Autodesk Inventor part; units mm, degrees
(part 2 of 4)
  arc A608 (10.5835, 25.1123) -> (10.4066, 24.8539) centre (14.8434, 22.0065) ccw
  arc A609 (10.8252, 25.4234) -> (10.5835, 25.1123) centre (15.7615, 21.3378) ccw
  arc A610 (11.147, 25.7878) -> (10.8252, 25.4234) centre (16.6706, 20.5861) ccw
  arc A611 (9.9958, 26.1618) -> (9.6113, 26.2702) centre (4.2393, 6.4866) ccw
  arc A612 (10.0419, 25.6779) -> (9.9958, 26.1618) centre (2.4697, 25.2002) ccw
  arc A613 (10.0547, 25.2841) -> (10.0419, 25.6779) centre (3.647, 25.2741) ccw
  arc A614 (10.4066, 24.8539) -> (10.0459, 24.9711) centre (4.2393, 6.4866) ccw
  arc A615 (10.0459, 24.9711) -> (10.0547, 25.2841) centre (4.7827, 25.2754) ccw
  arc A616 (9.1026, 25.5526) -> (8.9465, 25.2811) centre (13.5931, 22.7906) ccw
  arc A617 (9.3192, 25.8817) -> (9.1026, 25.5526) centre (14.5608, 22.1961) ccw
  arc A618 (9.6113, 26.2702) -> (9.3192, 25.8817) centre (15.526, 21.5179) ccw
  arc A619 (8.4344, 26.5528) -> (8.0426, 26.6307) centre (4.2393, 6.4866) ccw
  arc A620 (8.5183, 26.074) -> (8.4344, 26.5528) centre (1.0069, 25.0037) ccw
  arc A621 (8.5619, 25.6824) -> (8.5183, 26.074) centre (2.1747, 25.1697) ccw
  arc A622 (8.9465, 25.2811) -> (8.5777, 25.3697) centre (4.2393, 6.4866) ccw
  arc A623 (8.5777, 25.3697) -> (8.5619, 25.6824) centre (3.3069, 25.2601) ccw
  arc A624 (7.5917, 25.8754) -> (7.4574, 25.5925) centre (12.285, 23.4742) ccw
  arc A625 (7.7818, 26.2205) -> (7.5917, 25.8754) centre (13.2964, 22.9575) ccw
  arc A626 (8.0426, 26.6307) -> (7.7818, 26.2205) centre (14.3119, 22.3571) ccw
  arc A627 (6.8471, 26.8201) -> (6.4504, 26.867) centre (4.2393, 6.4866) ccw
  arc A628 (6.9683, 26.3493) -> (6.8471, 26.8201) centre (-0.436, 24.693) ccw
  arc A629 (7.0425, 25.9624) -> (6.9683, 26.3493) centre (0.7152, 24.9501) ccw
  arc A630 (7.4574, 25.5925) -> (7.0828, 25.6518) centre (4.2393, 6.4866) ccw
  arc A631 (7.0828, 25.6518) -> (7.0425, 25.9624) centre (1.8368, 25.1291) ccw
  arc A632 (6.0601, 26.0787) -> (5.9484, 25.7861) centre (10.9274, 24.0531) ccw
  arc A633 (6.2226, 26.4376) -> (6.0601, 26.0787) centre (11.9762, 23.6173) ccw
  arc A634 (6.4504, 26.867) -> (6.2226, 26.4376) centre (13.0356, 23.0985) ccw
  arc A635 (5.2437, 26.962) -> (4.8445, 26.9777) centre (4.2393, 6.4866) ccw
  arc A636 (5.4015, 26.5022) -> (5.2437, 26.962) centre (-1.85, 24.27) ccw
  arc A637 (5.5058, 26.1223) -> (5.4015, 26.5022) centre (-0.7225, 24.6167) ccw
  arc A638 (5.9484, 25.7861) -> (5.5703, 25.8158) centre (4.2393, 6.4866) ccw
  arc A639 (5.5703, 25.8158) -> (5.5058, 26.1223) centre (0.3816, 24.8831) ccw
  circle A640 centre (4.2393, 6.4866) radius 18.25
  circle A641 centre (4.2393, 6.4866) radius 4 construction
  circle A642 centre (4.2393, 6.4866) radius 20.5 construction
  circle A643 centre (4.2393, 6.4866) radius 2
  point P0 (0, 0)
  point P1 (0, 0)
  point P2 (4.2393, 28.9866)
  point P3 (2.474, 28.9173)
  point P4 (0.7195, 28.7096)
  point P5 (-1.0132, 28.3649)
  point P6 (-2.7136, 27.8854)
  point P7 (-4.3711, 27.2739)
  point P8 (-5.9755, 26.5343)
  point P9 (-7.5169, 25.671)
  point P10 (-8.9859, 24.6895)
  point P11 (-10.3733, 23.5958)
  point P12 (-11.6706, 22.3965)
  point P13 (-12.8698, 21.0992)
  point P14 (-13.9636, 19.7118)
  point P15 (-14.9451, 18.2428)
  point P16 (-15.8083, 16.7014)
  point P17 (-16.548, 15.097)
  point P18 (-17.1595, 13.4395)
  point P19 (-17.639, 11.7391)
  point P20 (-17.9837, 10.0064)
  point P21 (-18.1913, 8.252)
  point P22 (-18.2607, 6.4866)
  point P23 (-18.1913, 4.7213)
  point P24 (-17.9837, 2.9668)
  point P25 (-17.639, 1.2341)
  point P26 (-17.1595, -0.4663)
  point P27 (-16.548, -2.1238)
  point P28 (-15.8083, -3.7282)
  point P29 (-14.9451, -5.2696)
  point P30 (-13.9636, -6.7385)
  point P31 (-12.8698, -8.126)
  point P32 (-11.6706, -9.4233)
  point P33 (-10.3733, -10.6225)
  point P34 (-8.9859, -11.7163)
  point P35 (-7.5169, -12.6978)
  point P36 (-5.9755, -13.561)
  point P37 (-4.3711, -14.3007)
  point P38 (-2.7136, -14.9121)
  point P39 (-1.0132, -15.3917)
  point P40 (0.7195, -15.7364)
  point P41 (2.474, -15.944)
  point P42 (4.2393, -16.0134)
  point P43 (6.0046, -15.944)
  point P44 (7.7591, -15.7364)
  point P45 (9.4918, -15.3917)
  point P46 (11.1922, -14.9121)
  point P47 (12.8497, -14.3007)
  point P48 (14.4541, -13.561)
  point P49 (15.9955, -12.6978)
  point P50 (17.4645, -11.7163)
  point P51 (18.8519, -10.6225)
  point P52 (20.1492, -9.4233)
  point P53 (21.3484, -8.126)
  point P54 (22.4422, -6.7385)
  point P55 (23.4237, -5.2696)
  point P56 (24.287, -3.7282)
  point P57 (25.0266, -2.1238)
  point P58 (25.6381, -0.4663)
  point P59 (26.1176, 1.2341)
  point P60 (26.4623, 2.9668)
  point P61 (26.6699, 4.7213)
  point P62 (26.7393, 6.4866)
  point P63 (26.6699, 8.252)
  point P64 (26.4623, 10.0064)
  point P65 (26.1176, 11.7391)
  point P66 (25.6381, 13.4395)
  point P67 (25.0266, 15.097)
  point P68 (24.287, 16.7014)
  point P69 (23.4237, 18.2428)
  point P70 (22.4422, 19.7118)
  point P71 (21.3484, 21.0992)
  point P72 (20.1492, 22.3965)
  point P73 (18.8519, 23.5958)
  point P74 (17.4645, 24.6895)
  point P75 (15.9955, 25.671)
  point P76 (14.4541, 26.5343)
  point P77 (12.8497, 27.2739)
  point P78 (11.1922, 27.8854)
  point P79 (9.4918, 28.3649)
  point P80 (7.7591, 28.7096)
  point P81 (6.0046, 28.9173)
  point P82 (6.9688, 26.347)
  point P83 (6.8471, 26.8201)
  point P84 (6.4504, 26.867)
  point P85 (6.2215, 26.4355)
  point P86 (6.059, 26.0761)
  point P87 (5.9484, 25.7861)
  point P88 (5.5703, 25.8158)
  point P89 (5.5065, 26.1196)
  point P90 (5.4022, 26.5)
  point P91 (5.2437, 26.962)
  point P92 (4.8445, 26.9777)
  point P93 (4.6502, 26.5295)
  point P94 (4.5165, 26.1585)
  point P95 (4.4289, 25.8607)
  point P96 (4.0497, 25.8607)
  point P97 (3.9622, 26.1585)
  point P98 (3.8284, 26.5295)
  point P99 (3.6341, 26.9777)
  point P100 (3.2349, 26.962)
  point P101 (3.0764, 26.5)
  point P102 (2.9722, 26.1196)
  point P103 (2.9083, 25.8158)
  point P104 (2.5302, 25.7861)
  point P105 (2.4196, 26.0761)
  point P106 (2.2571, 26.4355)
  point P107 (2.0283, 26.867)
  point P108 (1.6316, 26.8201)
  point P109 (1.5098, 26.347)
  point P110 (1.4357, 25.9597)
  point P111 (1.3958, 25.6518)
  point P112 (1.0212, 25.5925)
  point P113 (0.8882, 25.8729)
  point P114 (0.698, 26.2185)
  point P115 (0.436, 26.6307)
  point P116 (0.0443, 26.5528)
  point P117 (-0.04, 26.0716)
  point P118 (-0.0835, 25.6797)
  point P119 (-0.0991, 25.3697)
  point P120 (-0.4679, 25.2811)
  point P121 (-0.6225, 25.5503)
  point P122 (-0.8392, 25.8798)
  point P123 (-1.1327, 26.2702)
  point P124 (-1.5172, 26.1618)
  point P125 (-1.5635, 25.6755)
  point P126 (-1.5761, 25.2813)
  point P127 (-1.5673, 24.9711)
  point P128 (-1.928, 24.8539)
  point P129 (-2.1032, 25.11)
  point P130 (-2.3451, 25.4216)
  point P131 (-2.6684, 25.7878)
  point P132 (-3.0431, 25.6495)
  point P133 (-3.0511, 25.1611)
  point P134 (-3.0327, 24.7671)
  point P135 (-2.9996, 24.4585)
  point P136 (-3.35, 24.3134)
  point P137 (-3.5448, 24.555)
  point P138 (-3.8104, 24.8466)
  point P139 (-4.1614, 25.1863)
  point P140 (-4.5242, 25.0191)
  point P141 (-4.4938, 24.5315)
  point P142 (-4.4446, 24.1402)
  point P143 (-4.3874, 23.8351)
  point P144 (-4.7253, 23.663)
  point P145 (-4.9385, 23.8886)
  point P146 (-5.2261, 24.1584)
  point P147 (-5.6027, 24.4695)
  point P148 (-5.9512, 24.2743)
  point P149 (-5.8827, 23.7907)
  point P150 (-5.8029, 23.4045)
  point P151 (-5.7219, 23.1048)
  point P152 (-6.0453, 22.9067)
  point P153 (-6.2755, 23.1148)
  point P154 (-6.5834, 23.3613)
  point P155 (-6.9833, 23.6419)
  point P156 (-7.3154, 23.42)
  point P157 (-7.2092, 22.9432)
  point P158 (-7.0993, 22.5644)
  point P159 (-6.9951, 22.272)
  point P160 (-7.3019, 22.0491)
  point P161 (-7.5477, 22.2386)
  point P162 (-7.874, 22.4601)
  point P163 (-8.2947, 22.7085)
  point P164 (-8.6084, 22.4612)
  point P165 (-8.465, 21.9942)
  point P166 (-8.3258, 21.6252)
  point P167 (-8.199, 21.3419)
  point P168 (-8.4873, 21.0956)
  point P169 (-8.7473, 21.2652)
  point P170 (-9.09, 21.4605)
  point P171 (-9.5288, 21.6751)
  point P172 (-9.8221, 21.4039)
  point P173 (-9.6426, 20.9496)
  point P174 (-9.4748, 20.5927)
  point P175 (-9.3261, 20.3202)
  point P176 (-9.5943, 20.0521)
  point P177 (-9.8668, 20.2008)
  point P178 (-10.2237, 20.3685)
  point P179 (-10.678, 20.548)
  point P180 (-10.9492, 20.2547)
  point P181 (-10.7345, 19.8159)
  point P182 (-10.5393, 19.4732)
  point P183 (-10.3697, 19.2133)
  point P184 (-10.616, 18.9249)
  point P185 (-10.8993, 19.0517)
  point P186 (-11.2683, 19.191)
  point P187 (-11.7353, 19.3343)
  point P188 (-11.9826, 19.0206)
  point P189 (-11.7342, 18.6)
  point P190 (-11.5127, 18.2737)
  point P191 (-11.3232, 18.0278)
  point P192 (-11.5461, 17.721)
  point P193 (-11.8385, 17.8252)
  point P194 (-12.2173, 17.9351)
  point P195 (-12.694, 18.0413)
  point P196 (-12.916, 17.7092)
  point P197 (-12.6353, 17.3094)
  point P198 (-12.3889, 17.0015)
  point P199 (-12.1807, 16.7712)
  dimension "d4" = 360
  dimension "d23" = 8
  dimension "d25" = 4
  constraints: 1280 point on circle, 643 centre point, 5 coincident, 2642 other
  measures "d23" diameter of A641
  measures "d25" diameter of A643
extrude "押し出し7" add sketch "スケッチ1" along normal blind 3 contours A1 A2 A635 A636 A637 A639 A638 A632 A633 A634 A627 A628 A629 A631 A630 A624 A625 A626 A619 A620 A621 A623 A622 A616 A617 A618 A611 A612 A613 A615 A614 A608 A609 A610 A603 A604 A605 A607 A606 A600 A601 A602 A595 A596 A597 A599 A598 A592 A593 A594 A587 A588 A589 A591 A590 A584 A585 A586 A579 A580 A581 A583 A582 A576 A577 A578 A571 A572 A573 A575 A574 A568 A569 A570 A563 A564 A565 A567 A566 A560 A561 A562 A555 A556 A557 A559 A558 A552 A553 A554 A547 A548 A549 A551 A550 A544 A545 A546 A539 A540 A541 A543 A542 A536 A537 A538 A531 A532 A533 A535 A534 A528 A529 A530 A523 A524 A525 A527 A526 A520 A521 A522 A515 A516 A517 A519 A518 A512 A513 A514 A507 A508 A509 A511 A510 A504 A505 A506 A499 A500 A501 A503 A502 A496 A497 A498 A491 A492 A493 A495 A494 A488 A489 A490 A483 A484 A485 A487 A486 A480 A481 A482 A475 A476 A477 A479 A478 A472 A473 A474 A467 A468 A469 A471 A470 A464 A465 A466 A459 A460 A461 A463 A462 A456 A457 A458 A451 A452 A453 A455 A454 A448 A449 A450 A443 A444 A445 A447 A446 A440 A441 A442 A435 A436 A437 A439 A438 A432 A433 A434 A427 A428 A429 A431 A430 A424 A425 A426 A419 A420 A421 A423 A422 A416 A417 A418 A411 A412 A413 A415 A414 A408 A409 A410 A403 A404 A405 A407 A406 A400 A401 A402 A395 A396 A397 A399 A398 A392 A393 A394 A387 A388 A389 A391 A390 A384 A385 A386 A379 A380 A381 A383 A382 A376 A377 A378 A371 A372 A373 A375 A374 A368 A369 A370 A363 A364 A365 A367 A366 A360 A361 A362 A355 A356 A357 A359 A358 A352 A353 A354 A347 A348 A349 A351 A350 A344 A345 A346 A339 A340 A341 A343 A342 A336 A337 A338 A331 A332 A333 A335 A334 A328 A329 A330 A323 A324 A325 A327 A326 A320 A321 A322 A315 A316 A317 A319 A318 A312 A313 A314 A307 A308 A309 A311 A310 A304 A305 A306 A299 A300 A301 A303 A302 A296 A297 A298 A291 A292 A293 A295 A294 A288 A289 A290 A283 A284 A285 A287 A286 A280 A281 A282 A275 A276 A277 A279 A278 A272 A273 A274 A267 A268 A269 A271 A270 A264 A265 A266 A259 A260 A261 A263 A262 A256 A257 A258 A251 A252 A253 A255 A254 A248 A249 A250 A243 A244 A245 A247 A246 A240 A241 A242 A235 A236 A237 A239 A238 A232 A233 A234 A227 A228 A229 A231 A230 A224 A225 A226 A219 A220 A221 A223 A222 A216 A217 A218 A211 A212 A213 A215 A214 A208 A209 A210 A203 A204 A205 A207 A206 A200 A201 A202 A195 A196 A197 A199 A198 A192 A193 A194 A187 A188 A189 A191 A190 A184 A185 A186 A179 A180 A181 A183 A182 A176 A177 A178 A171 A172 A173 A175 A174 A168 A169 A170 A163 A164 A165 A167 A166 A160 A161 A162 A155 A156 A157 A159 A158 A152 A153 A154 A147 A148 A149 A151 A150 A144 A145 A146 A139 A140 A141 A143 A142 A136 A137 A138 A131 A132 A133 A135 A134 A128 A129 A130 A123 A124 A125 A127 A126 A120 A121 A122 A115 A116 A117 A119 A118 A112 A113 A114 A107 A108 A109 A111 A110 A104 A105 A106 A99 A100 A101 A103 A102 A96 A97 A98 A91 A92 A93 A95 A94 A88 A89 A90 A83 A84 A85 A87 A86 A80 A81 A82 A75 A76 A77 A79 A78 A72 A73 A74 A67 A68 A69 A71 A70 A64 A65 A66 A59 A60 A61 A63 A62 A56 A57 A58 A51 A52 A53 A55 A54 A48 A49 A50 A43 A44 A45 A47 A46 A40 A41 A42 A35 A36 A37 A39 A38 A32 A33 A34 A27 A28 A29 A31 A30 A24 A25 A26 A19 A20 A21 A23 A22 A16 A17 A18 A11 A12 A13 A15 A14 A8 A9 A10 A7 A5 A4 A3 A6 A0 | A640
sketch "スケッチ2" plane through (0, 0, 3) normal (0, 0, 1) x (1, 0, 0)
  arc A0 (-6.5853, 23.3627) -> (-6.9833, 23.6419) centre (-11.1399, 17.2945) ccw
  arc A1 (-6.9833, 23.6419) -> (-7.3154, 23.42) centre (4.2393, 6.4866) ccw
  arc A2 (-7.3154, 23.42) -> (-7.2097, 22.9455) centre (0.1395, 24.8311) ccw
  arc A3 (-7.2097, 22.9455) -> (-7.1002, 22.567) centre (-1.003, 24.5376) ccw
  arc A4 (-7.1002, 22.567) -> (-6.9951, 22.272) centre (-2.0836, 24.1879) ccw
  arc A5 (-6.9951, 22.272) -> (-7.3019, 22.0491) centre (4.2393, 6.4866) ccw
  arc A6 (-7.3019, 22.0491) -> (-7.55, 22.2402) centre (-10.6417, 17.97) ccw
  arc A7 (-7.55, 22.2402) -> (-7.876, 22.4614) centre (-11.3083, 17.0504) ccw
  arc A8 (-7.876, 22.4614) -> (-8.2947, 22.7085) centre (-11.9405, 16.0545) ccw
  arc A9 (-8.2947, 22.7085) -> (-8.6084, 22.4612) centre (4.2393, 6.4866) ccw
  arc A10 (-8.6084, 22.4612) -> (-8.4658, 21.9965) centre (-1.2871, 24.4529) ccw
  arc A11 (-8.4658, 21.9965) -> (-8.3269, 21.6278) centre (-2.4031, 24.0707) ccw
  arc A12 (-8.3269, 21.6278) -> (-8.199, 21.3419) centre (-3.4529, 23.6372) ccw
  arc A13 (-8.199, 21.3419) -> (-8.4873, 21.0956) centre (4.2393, 6.4866) ccw
  arc A14 (-8.4873, 21.0956) -> (-8.7497, 21.2667) centre (-11.4968, 16.7671) ccw
  arc A15 (-8.7497, 21.2667) -> (-9.0921, 21.4616) centre (-12.0892, 15.798) ccw
  arc A16 (-9.0921, 21.4616) -> (-9.5288, 21.6751) centre (-12.6413, 14.7556) ccw
  arc A17 (-9.5288, 21.6751) -> (-9.8221, 21.4039) centre (4.2393, 6.4866) ccw
  arc A18 (-9.8221, 21.4039) -> (-9.6435, 20.9518) centre (-2.6797, 23.964) ccw
  arc A19 (-9.6435, 20.9518) -> (-9.4761, 20.5952) centre (-3.7622, 23.4953) ccw
  arc A20 (-9.4761, 20.5952) -> (-9.3261, 20.3202) centre (-4.7748, 22.9808) ccw
  arc A21 (-9.3261, 20.3202) -> (-9.5943, 20.0521) centre (4.2393, 6.4866) ccw
  arc A22 (-9.5943, 20.0521) -> (-9.8693, 20.202) centre (-12.2549, 15.5007) ccw
  arc A23 (-9.8693, 20.202) -> (-10.2259, 20.3695) centre (-12.7694, 14.4882) ccw
  arc A24 (-10.2259, 20.3695) -> (-10.678, 20.548) centre (-13.238, 13.4056) ccw
  arc A25 (-10.678, 20.548) -> (-10.9492, 20.2547) centre (4.2393, 6.4866) ccw
  arc A26 (-10.9492, 20.2547) -> (-10.7357, 19.818) centre (-4.0296, 23.3672) ccw
  arc A27 (-10.7357, 19.818) -> (-10.5408, 19.4756) centre (-5.0721, 22.8151) ccw
  arc A28 (-10.5408, 19.4756) -> (-10.3697, 19.2133) centre (-6.0411, 22.2227) ccw
  arc A29 (-10.3697, 19.2133) -> (-10.616, 18.9249) centre (4.2393, 6.4866) ccw
  arc A30 (-10.616, 18.9249) -> (-10.9019, 19.0528) centre (-12.9113, 14.1788) ccw
  arc A31 (-10.9019, 19.0528) -> (-11.2705, 19.1917) centre (-13.3447, 13.129) ccw
  arc A32 (-11.2705, 19.1917) -> (-11.7353, 19.3343) centre (-13.727, 12.0131) ccw
  arc A33 (-11.7353, 19.3343) -> (-11.9826, 19.0206) centre (4.2393, 6.4866) ccw
  arc A34 (-11.9826, 19.0206) -> (-11.7355, 18.602) centre (-5.3286, 22.6664) ccw
  arc A35 (-11.7355, 18.602) -> (-11.5143, 18.2759) centre (-6.3245, 22.0342) ccw
  arc A36 (-11.5143, 18.2759) -> (-11.3232, 18.0278) centre (-7.2441, 21.3676) ccw
  arc A37 (-11.3232, 18.0278) -> (-11.5461, 17.721) centre (4.2393, 6.4866) ccw
  arc A38 (-11.5461, 17.721) -> (-11.8411, 17.8261) centre (-13.4619, 12.8095) ccw
  arc A39 (-11.8411, 17.8261) -> (-12.2196, 17.9357) centre (-13.8117, 11.7289) ccw
  arc A40 (-12.2196, 17.9357) -> (-12.694, 18.0413) centre (-14.1052, 10.5864) ccw
  arc A41 (-12.694, 18.0413) -> (-12.916, 17.7092) centre (4.2393, 6.4866) ccw
  arc A42 (-12.916, 17.7092) -> (-12.6368, 17.3113) centre (-6.5685, 21.8658) ccw
  arc A43 (-12.6368, 17.3113) -> (-12.3907, 17.0036) centre (-7.5118, 21.1574) ccw
  arc A44 (-12.3907, 17.0036) -> (-12.1807, 16.7712) centre (-8.3762, 20.4208) ccw
  arc A45 (-12.1807, 16.7712) -> (-12.3789, 16.4479) centre (4.2393, 6.4866) ccw
  arc A46 (-12.3789, 16.4479) -> (-12.6812, 16.5295) centre (-13.9035, 11.4012) ccw
  arc A47 (-12.6812, 16.5295) -> (-13.0671, 16.609) centre (-14.1674, 10.2965) ccw
  arc A48 (-13.0671, 16.609) -> (-13.5484, 16.6771) centre (-14.3703, 9.1345) ccw
  arc A49 (-13.5484, 16.6771) -> (-13.7436, 16.3286) centre (4.2393, 6.4866) ccw
  arc A50 (-13.7436, 16.3286) -> (-13.434, 15.9538) centre (-7.7419, 20.9705) ccw
  arc A51 (-13.434, 15.9538) -> (-13.1646, 15.6664) centre (-8.6266, 20.1902) ccw
  arc A52 (-13.1646, 15.6664) -> (-12.937, 15.4512) centre (-9.4306, 19.388) ccw
  arc A53 (-12.937, 15.4512) -> (-13.1092, 15.1133) centre (4.2393, 6.4866) ccw
  arc A54 (-13.1092, 15.1133) -> (-13.417, 15.171) centre (-14.2331, 9.9626) ccw
  arc A55 (-13.417, 15.171) -> (-13.8079, 15.22) centre (-14.4095, 8.8406) ccw
  arc A56 (-13.8079, 15.22) -> (-14.2931, 15.2501) centre (-14.5207, 7.6662) ccw
  arc A57 (-14.2931, 15.2501) -> (-14.4604, 14.8874) centre (4.2393, 6.4866) ccw
  arc A58 (-14.4604, 14.8874) -> (-14.1223, 14.538) centre (-8.8413, 19.9858) ccw
  arc A59 (-14.1223, 14.538) -> (-13.8312, 14.2726) centre (-9.6621, 19.1385) ccw
  arc A60 (-13.8312, 14.2726) -> (-13.5874, 14.076) centre (-10.4007, 18.2757) ccw
  arc A61 (-13.5874, 14.076) -> (-13.7326, 13.7256) centre (4.2393, 6.4866) ccw
  arc A62 (-13.7326, 13.7256) -> (-14.044, 13.7589) centre (-14.4489, 8.5025) ccw
  arc A63 (-14.044, 13.7589) -> (-14.4375, 13.7771) centre (-14.5367, 7.3701) ccw
  arc A64 (-14.4375, 13.7771) -> (-14.9236, 13.7691) centre (-14.5554, 6.1907) ccw
  arc A65 (-14.9236, 13.7691) -> (-15.0618, 13.3943) centre (4.2393, 6.4866) ccw
  arc A66 (-15.0618, 13.3943) -> (-14.6974, 13.0725) centre (-9.8601, 18.9179) ccw
  arc A67 (-14.6974, 13.0725) -> (-14.3864, 12.8308) centre (-10.6119, 18.0089) ccw
  arc A68 (-14.3864, 12.8308) -> (-14.1279, 12.6539) centre (-11.2805, 17.0907) ccw
  arc A69 (-14.1279, 12.6539) -> (-14.2451, 12.2932) centre (4.2393, 6.4866) ccw
  arc A70 (-14.2451, 12.2932) -> (-14.5582, 12.302) centre (-14.5494, 7.0301) ccw
  arc A71 (-14.5582, 12.302) -> (-14.9519, 12.2893) centre (-14.5482, 5.8943) ccw
  arc A72 (-14.9519, 12.2893) -> (-15.4359, 12.2431) centre (-14.4743, 4.717) ccw
  arc A73 (-15.4359, 12.2431) -> (-15.5443, 11.8587) centre (4.2393, 6.4866) ccw
  arc A74 (-15.5443, 11.8587) -> (-15.1558, 11.5665) centre (-10.792, 17.7733) ccw
  arc A75 (-15.1558, 11.5665) -> (-14.8267, 11.3499) centre (-11.4701, 16.8081) ccw
  arc A76 (-14.8267, 11.3499) -> (-14.5552, 11.1938) centre (-12.0647, 15.8404) ccw
  arc A77 (-14.5552, 11.1938) -> (-14.6437, 10.825) centre (4.2393, 6.4866) ccw
  arc A78 (-14.6437, 10.825) -> (-14.9565, 10.8092) centre (-14.5342, 5.5542) ccw
  arc A79 (-14.9565, 10.8092) -> (-15.3481, 10.7656) centre (-14.4438, 4.422) ccw
  arc A80 (-15.3481, 10.7656) -> (-15.8269, 10.6817) centre (-14.2777, 3.2542) ccw
  arc A81 (-15.8269, 10.6817) -> (-15.9048, 10.2899) centre (4.2393, 6.4866) ccw
  arc A82 (-15.9048, 10.2899) -> (-15.4946, 10.0291) centre (-11.6312, 16.5592) ccw
  arc A83 (-15.4946, 10.0291) -> (-15.1495, 9.839) centre (-12.2315, 15.5438) ccw
  arc A84 (-15.1495, 9.839) -> (-14.8666, 9.7047) centre (-12.7483, 14.5323) ccw
  arc A85 (-14.8666, 9.7047) -> (-14.9259, 9.3301) centre (4.2393, 6.4866) ccw
  arc A86 (-14.9259, 9.3301) -> (-15.2365, 9.2898) centre (-14.4031, 4.0842) ccw
  arc A87 (-15.2365, 9.2898) -> (-15.6234, 9.2156) centre (-14.2242, 2.9626) ccw
  arc A88 (-15.6234, 9.2156) -> (-16.0942, 9.0944) centre (-13.967, 1.8113) ccw
  arc A89 (-16.0942, 9.0944) -> (-16.1411, 8.6977) centre (4.2393, 6.4866) ccw
  arc A90 (-16.1411, 8.6977) -> (-15.7117, 8.4699) centre (-12.3726, 15.2829) ccw
  arc A91 (-15.7117, 8.4699) -> (-15.3527, 8.3074) centre (-12.8914, 14.2235) ccw
  arc A92 (-15.3527, 8.3074) -> (-15.0602, 8.1957) centre (-13.3272, 13.1747) ccw
  arc A93 (-15.0602, 8.1957) -> (-15.0899, 7.8177) centre (4.2393, 6.4866) ccw
  arc A94 (-15.0899, 7.8177) -> (-15.3964, 7.7531) centre (-14.1572, 2.6289) ccw
  arc A95 (-15.3964, 7.7531) -> (-15.7763, 7.6488) centre (-13.8908, 1.5248) ccw
  arc A96 (-15.7763, 7.6488) -> (-16.2361, 7.491) centre (-13.5441, 0.3973) ccw
  arc A97 (-16.2361, 7.491) -> (-16.2518, 7.0918) centre (4.2393, 6.4866) ccw
  arc A98 (-16.2518, 7.0918) -> (-15.8058, 6.8984) centre (-13.0115, 13.9525) ccw
  arc A99 (-15.8058, 6.8984) -> (-15.4352, 6.7646) centre (-13.4456, 12.8556) ccw
  arc A100 (-15.4352, 6.7646) -> (-15.1348, 6.6762) centre (-13.7978, 11.7758) ccw
  arc A101 (-15.1348, 6.6762) -> (-15.1348, 6.297) centre (4.2393, 6.4866) ccw
  arc A102 (-15.1348, 6.297) -> (-15.4352, 6.2086) centre (-13.7978, 1.1974) ccw
  arc A103 (-15.4352, 6.2086) -> (-15.8058, 6.0748) centre (-13.4456, 0.1176) ccw
  arc A104 (-15.8058, 6.0748) -> (-16.2518, 5.8814) centre (-13.0115, -0.9792) ccw
  arc A105 (-16.2518, 5.8814) -> (-16.2361, 5.4823) centre (4.2393, 6.4866) ccw
  arc A106 (-16.2361, 5.4823) -> (-15.7763, 5.3244) centre (-13.5441, 12.576) ccw
  arc A107 (-15.7763, 5.3244) -> (-15.3964, 5.2201) centre (-13.8908, 11.4485) ccw
  arc A108 (-15.3964, 5.2201) -> (-15.0899, 5.1556) centre (-14.1572, 10.3443) ccw
  arc A109 (-15.0899, 5.1556) -> (-15.0602, 4.7775) centre (4.2393, 6.4866) ccw
  arc A110 (-15.0602, 4.7775) -> (-15.3527, 4.6658) centre (-13.3272, -0.2015) ccw
  arc A111 (-15.3527, 4.6658) -> (-15.7117, 4.5034) centre (-12.8914, -1.2503) ccw
  arc A112 (-15.7117, 4.5034) -> (-16.1411, 4.2756) centre (-12.3726, -2.3097) ccw
  arc A113 (-16.1411, 4.2756) -> (-16.0942, 3.8789) centre (4.2393, 6.4866) ccw
  arc A114 (-16.0942, 3.8789) -> (-15.6234, 3.7576) centre (-13.967, 11.1619) ccw
  arc A115 (-15.6234, 3.7576) -> (-15.2365, 3.6834) centre (-14.2242, 10.0107) ccw
  arc A116 (-15.2365, 3.6834) -> (-14.9259, 3.6431) centre (-14.4031, 8.8891) ccw
  arc A117 (-14.9259, 3.6431) -> (-14.8666, 3.2686) centre (4.2393, 6.4866) ccw
  arc A118 (-14.8666, 3.2686) -> (-15.1495, 3.1343) centre (-12.7483, -1.5591) ccw
  arc A119 (-15.1495, 3.1343) -> (-15.4946, 2.9442) centre (-12.2315, -2.5705) ccw
  arc A120 (-15.4946, 2.9442) -> (-15.9048, 2.6834) centre (-11.6312, -3.5859) ccw
  arc A121 (-15.9048, 2.6834) -> (-15.8269, 2.2916) centre (4.2393, 6.4866) ccw
  arc A122 (-15.8269, 2.2916) -> (-15.3481, 2.2076) centre (-14.2777, 9.7191) ccw
  arc A123 (-15.3481, 2.2076) -> (-14.9565, 2.164) centre (-14.4438, 8.5512) ccw
  arc A124 (-14.9565, 2.164) -> (-14.6437, 2.1482) centre (-14.5342, 7.419) ccw
  arc A125 (-14.6437, 2.1482) -> (-14.5552, 1.7794) centre (4.2393, 6.4866) ccw
  arc A126 (-14.5552, 1.7794) -> (-14.8267, 1.6234) centre (-12.0647, -2.8671) ccw
  arc A127 (-14.8267, 1.6234) -> (-15.1558, 1.4068) centre (-11.4701, -3.8349) ccw
  arc A128 (-15.1558, 1.4068) -> (-15.5443, 1.1146) centre (-10.792, -4.8001) ccw
  arc A129 (-15.5443, 1.1146) -> (-15.4359, 0.7301) centre (4.2393, 6.4866) ccw
  arc A130 (-15.4359, 0.7301) -> (-14.9519, 0.684) centre (-14.4743, 8.2563) ccw
  arc A131 (-14.9519, 0.684) -> (-14.5582, 0.6713) centre (-14.5482, 7.079) ccw
  arc A132 (-14.5582, 0.6713) -> (-14.2451, 0.6801) centre (-14.5494, 5.9432) ccw
  arc A133 (-14.2451, 0.6801) -> (-14.1279, 0.3194) centre (4.2393, 6.4866) ccw
  arc A134 (-14.1279, 0.3194) -> (-14.3864, 0.1425) centre (-11.2805, -4.1175) ccw
  arc A135 (-14.3864, 0.1425) -> (-14.6974, -0.0993) centre (-10.6119, -5.0356) ccw
  arc A136 (-14.6974, -0.0993) -> (-15.0618, -0.4211) centre (-9.8601, -5.9446) ccw
  arc A137 (-15.0618, -0.4211) -> (-14.9236, -0.7958) centre (4.2393, 6.4866) ccw
  arc A138 (-14.9236, -0.7958) -> (-14.4375, -0.8038) centre (-14.5554, 6.7826) ccw
  arc A139 (-14.4375, -0.8038) -> (-14.044, -0.7856) centre (-14.5367, 5.6031) ccw
  arc A140 (-14.044, -0.7856) -> (-13.7326, -0.7523) centre (-14.4489, 4.4707) ccw
  arc A141 (-13.7326, -0.7523) -> (-13.5874, -1.1027) centre (4.2393, 6.4866) ccw
  arc A142 (-13.5874, -1.1027) -> (-13.8312, -1.2993) centre (-10.4007, -5.3025) ccw
  arc A143 (-13.8312, -1.2993) -> (-14.1223, -1.5647) centre (-9.6621, -6.1653) ccw
  arc A144 (-14.1223, -1.5647) -> (-14.4604, -1.9141) centre (-8.8413, -7.0125) ccw
  arc A145 (-14.4604, -1.9141) -> (-14.2931, -2.2769) centre (4.2393, 6.4866) ccw
  arc A146 (-14.2931, -2.2769) -> (-13.8079, -2.2467) centre (-14.5207, 5.307) ccw
  arc A147 (-13.8079, -2.2467) -> (-13.417, -2.1977) centre (-14.4095, 4.1327) ccw
  arc A148 (-13.417, -2.1977) -> (-13.1092, -2.1401) centre (-14.2331, 3.0107) ccw
  arc A149 (-13.1092, -2.1401) -> (-12.937, -2.478) centre (4.2393, 6.4866) ccw
  arc A150 (-12.937, -2.478) -> (-13.1646, -2.6931) centre (-9.4306, -6.4148) ccw
  arc A151 (-13.1646, -2.6931) -> (-13.434, -2.9806) centre (-8.6266, -7.217) ccw
  arc A152 (-13.434, -2.9806) -> (-13.7436, -3.3554) centre (-7.7419, -7.9972) ccw
  arc A153 (-13.7436, -3.3554) -> (-13.5484, -3.7039) centre (4.2393, 6.4866) ccw
  arc A154 (-13.5484, -3.7039) -> (-13.0671, -3.6358) centre (-14.3703, 3.8388) ccw
  arc A155 (-13.0671, -3.6358) -> (-12.6812, -3.5562) centre (-14.1674, 2.6768) ccw
  arc A156 (-12.6812, -3.5562) -> (-12.3789, -3.4746) centre (-13.9035, 1.5721) ccw
  arc A157 (-12.3789, -3.4746) -> (-12.1807, -3.798) centre (4.2393, 6.4866) ccw
  arc A158 (-12.1807, -3.798) -> (-12.3907, -4.0303) centre (-8.3762, -7.4475) ccw
  arc A159 (-12.3907, -4.0303) -> (-12.6368, -4.338) centre (-7.5118, -8.1842) ccw
  arc A160 (-12.6368, -4.338) -> (-12.916, -4.736) centre (-6.5685, -8.8926) ccw
  arc A161 (-12.916, -4.736) -> (-12.694, -5.0681) centre (4.2393, 6.4866) ccw
  arc A162 (-12.694, -5.0681) -> (-12.2196, -4.9624) centre (-14.1052, 2.3868) ccw
  arc A163 (-12.2196, -4.9624) -> (-11.8411, -4.8528) centre (-13.8117, 1.2443) ccw
  arc A164 (-11.8411, -4.8528) -> (-11.5461, -4.7478) centre (-13.4619, 0.1637) ccw
  arc A165 (-11.5461, -4.7478) -> (-11.3232, -5.0546) centre (4.2393, 6.4866) ccw
  arc A166 (-11.3232, -5.0546) -> (-11.5143, -5.3027) centre (-7.2441, -8.3944) ccw
  arc A167 (-11.5143, -5.3027) -> (-11.7355, -5.6287) centre (-6.3245, -9.0609) ccw
  arc A168 (-11.7355, -5.6287) -> (-11.9826, -6.0473) centre (-5.3286, -9.6932) ccw
  arc A169 (-11.9826, -6.0473) -> (-11.7353, -6.3611) centre (4.2393, 6.4866) ccw
  arc A170 (-11.7353, -6.3611) -> (-11.2705, -6.2185) centre (-13.727, 0.9602) ccw
  arc A171 (-11.2705, -6.2185) -> (-10.9019, -6.0795) centre (-13.3447, -0.1558) ccw
  arc A172 (-10.9019, -6.0795) -> (-10.616, -5.9516) centre (-12.9113, -1.2056) ccw
  arc A173 (-10.616, -5.9516) -> (-10.3697, -6.24) centre (4.2393, 6.4866) ccw
  arc A174 (-10.3697, -6.24) -> (-10.5408, -6.5023) centre (-6.0411, -9.2495) ccw
  arc A175 (-10.5408, -6.5023) -> (-10.7357, -6.8447) centre (-5.0721, -9.8418) ccw
  arc A176 (-10.7357, -6.8447) -> (-10.9492, -7.2815) centre (-4.0296, -10.394) ccw
  arc A177 (-10.9492, -7.2815) -> (-10.678, -7.5748) centre (4.2393, 6.4866) ccw
  arc A178 (-10.678, -7.5748) -> (-10.2259, -7.3962) centre (-13.238, -0.4324) ccw
  arc A179 (-10.2259, -7.3962) -> (-9.8693, -7.2288) centre (-12.7694, -1.5149) ccw
  arc A180 (-9.8693, -7.2288) -> (-9.5943, -7.0788) centre (-12.2549, -2.5275) ccw
  arc A181 (-9.5943, -7.0788) -> (-9.3261, -7.347) centre (4.2393, 6.4866) ccw
  arc A182 (-9.3261, -7.347) -> (-9.4761, -7.6219) centre (-4.7748, -10.0076) ccw
  arc A183 (-9.4761, -7.6219) -> (-9.6435, -7.9786) centre (-3.7622, -10.5221) ccw
  arc A184 (-9.6435, -7.9786) -> (-9.8221, -8.4307) centre (-2.6797, -10.9907) ccw
  arc A185 (-9.8221, -8.4307) -> (-9.5288, -8.7019) centre (4.2393, 6.4866) ccw
  arc A186 (-9.5288, -8.7019) -> (-9.0921, -8.4883) centre (-12.6413, -1.7823) ccw
  arc A187 (-9.0921, -8.4883) -> (-8.7497, -8.2934) centre (-12.0892, -2.8247) ccw
  arc A188 (-8.7497, -8.2934) -> (-8.4873, -8.1224) centre (-11.4968, -3.7938) ccw
  arc A189 (-8.4873, -8.1224) -> (-8.199, -8.3687) centre (4.2393, 6.4866) ccw
  arc A190 (-8.199, -8.3687) -> (-8.3269, -8.6545) centre (-3.4529, -10.664) ccw
  arc A191 (-8.3269, -8.6545) -> (-8.4658, -9.0232) centre (-2.4031, -11.0974) ccw
  arc A192 (-8.4658, -9.0232) -> (-8.6084, -9.488) centre (-1.2871, -11.4797) ccw
  arc A193 (-8.6084, -9.488) -> (-8.2947, -9.7353) centre (4.2393, 6.4866) ccw
  arc A194 (-8.2947, -9.7353) -> (-7.876, -9.4881) centre (-11.9405, -3.0813) ccw
  arc A195 (-7.876, -9.4881) -> (-7.55, -9.267) centre (-11.3083, -4.0772) ccw
  arc A196 (-7.55, -9.267) -> (-7.3019, -9.0759) centre (-10.6417, -4.9968) ccw
  arc A197 (-7.3019, -9.0759) -> (-6.9951, -9.2988) centre (4.2393, 6.4866) ccw
  arc A198 (-6.9951, -9.2988) -> (-7.1002, -9.5938) centre (-2.0836, -11.2146) ccw
  arc A199 (-7.1002, -9.5938) -> (-7.2097, -9.9722) centre (-1.003, -11.5644) ccw
  arc A200 (-7.2097, -9.9722) -> (-7.3154, -10.4467) centre (0.1395, -11.8579) ccw
  arc A201 (-7.3154, -10.4467) -> (-6.9833, -10.6687) centre (4.2393, 6.4866) ccw
  arc A202 (-6.9833, -10.6687) -> (-6.5853, -10.3895) centre (-11.1399, -4.3212) ccw
  arc A203 (-6.5853, -10.3895) -> (-6.2776, -10.1434) centre (-10.4315, -5.2644) ccw
  arc A204 (-6.2776, -10.1434) -> (-6.0453, -9.9334) centre (-9.6948, -6.1289) ccw
  arc A205 (-6.0453, -9.9334) -> (-5.7219, -10.1316) centre (4.2393, 6.4866) ccw
  arc A206 (-5.7219, -10.1316) -> (-5.8036, -10.4339) centre (-0.6753, -11.6561) ccw
  arc A207 (-5.8036, -10.4339) -> (-5.8831, -10.8198) centre (0.4294, -11.92) ccw
  arc A208 (-5.8831, -10.8198) -> (-5.9512, -11.3011) centre (1.5915, -12.123) ccw
  arc A209 (-5.9512, -11.3011) -> (-5.6027, -11.4963) centre (4.2393, 6.4866) ccw
  arc A210 (-5.6027, -11.4963) -> (-5.2279, -11.1867) centre (-10.2445, -5.4945) ccw
  arc A211 (-5.2279, -11.1867) -> (-4.9404, -10.9173) centre (-9.4643, -6.3793) ccw
  arc A212 (-4.9404, -10.9173) -> (-4.7253, -10.6897) centre (-8.6621, -7.1833) ccw
  arc A213 (-4.7253, -10.6897) -> (-4.3874, -10.8619) centre (4.2393, 6.4866) ccw
  arc A214 (-4.3874, -10.8619) -> (-4.445, -11.1697) centre (0.7634, -11.9858) ccw
  arc A215 (-4.445, -11.1697) -> (-4.4941, -11.5606) centre (1.8854, -12.1622) ccw
  arc A216 (-4.4941, -11.5606) -> (-4.5242, -12.0458) centre (3.0597, -12.2734) ccw
  arc A217 (-4.5242, -12.0458) -> (-4.1614, -12.213) centre (4.2393, 6.4866) ccw
  arc A218 (-4.1614, -12.213) -> (-3.8121, -11.875) centre (-9.2598, -6.594) ccw
  arc A219 (-3.8121, -11.875) -> (-3.5466, -11.5839) centre (-8.4126, -7.4148) ccw
  arc A220 (-3.5466, -11.5839) -> (-3.35, -11.3401) centre (-7.5498, -8.1534) ccw
  arc A221 (-3.35, -11.3401) -> (-2.9996, -11.4853) centre (4.2393, 6.4866) ccw
  arc A222 (-2.9996, -11.4853) -> (-3.033, -11.7966) centre (2.2234, -12.2016) ccw
  arc A223 (-3.033, -11.7966) -> (-3.0512, -12.1902) centre (3.3558, -12.2894) ccw
  arc A224 (-3.0512, -12.1902) -> (-3.0431, -12.6763) centre (4.5353, -12.3081) ccw
  arc A225 (-3.0431, -12.6763) -> (-2.6684, -12.8145) centre (4.2393, 6.4866) ccw
  arc A226 (-2.6684, -12.8145) -> (-2.3466, -12.4501) centre (-8.1919, -7.6128) ccw
  arc A227 (-2.3466, -12.4501) -> (-2.1048, -12.139) centre (-7.2829, -8.3646) ccw
  arc A228 (-2.1048, -12.139) -> (-1.928, -11.8806) centre (-6.3648, -9.0332) ccw
  arc A229 (-1.928, -11.8806) -> (-1.5673, -11.9978) centre (4.2393, 6.4866) ccw
  arc A230 (-1.5673, -11.9978) -> (-1.576, -12.3109) centre (3.6959, -12.3021) ccw
  arc A231 (-1.576, -12.3109) -> (-1.5633, -12.7046) centre (4.8317, -12.3009) ccw
  arc A232 (-1.5633, -12.7046) -> (-1.5172, -13.1886) centre (6.009, -12.227) ccw
  arc A233 (-1.5172, -13.1886) -> (-1.1327, -13.297) centre (4.2393, 6.4866) ccw
  arc A234 (-1.1327, -13.297) -> (-0.8405, -12.9085) centre (-7.0474, -8.5447) ccw
  arc A235 (-0.8405, -12.9085) -> (-0.6239, -12.5794) centre (-6.0822, -9.2228) ccw
  arc A236 (-0.6239, -12.5794) -> (-0.4679, -12.3079) centre (-5.1144, -9.8174) ccw
  arc A237 (-0.4679, -12.3079) -> (-0.0991, -12.3964) centre (4.2393, 6.4866) ccw
  arc A238 (-0.0991, -12.3964) -> (-0.0833, -12.7092) centre (5.1717, -12.2869) ccw
  arc A239 (-0.0833, -12.7092) -> (-0.0397, -13.1007) centre (6.3039, -12.1965) ccw
  arc A240 (-0.0397, -13.1007) -> (0.0443, -13.5796) centre (7.4718, -12.0304) ccw
  arc A241 (0.0443, -13.5796) -> (0.436, -13.6575) centre (4.2393, 6.4866) ccw
  arc A242 (0.436, -13.6575) -> (0.6968, -13.2473) centre (-5.8332, -9.3839) ccw
  arc A243 (0.6968, -13.2473) -> (0.887, -12.9022) centre (-4.8178, -9.9842) ccw
  arc A244 (0.887, -12.9022) -> (1.0212, -12.6193) centre (-3.8064, -10.501) ccw
  arc A245 (1.0212, -12.6193) -> (1.3958, -12.6786) centre (4.2393, 6.4866) ccw
  arc A246 (1.3958, -12.6786) -> (1.4361, -12.9891) centre (6.6418, -12.1558) ccw
  arc A247 (1.4361, -12.9891) -> (1.5103, -13.3761) centre (7.7634, -11.9769) ccw
  arc A248 (1.5103, -13.3761) -> (1.6316, -13.8468) centre (8.9146, -11.7197) ccw
  arc A249 (1.6316, -13.8468) -> (2.0283, -13.8938) centre (4.2393, 6.4866) ccw
  arc A250 (2.0283, -13.8938) -> (2.2561, -13.4644) centre (-4.557, -10.1253) ccw
  arc A251 (2.2561, -13.4644) -> (2.4185, -13.1054) centre (-3.4976, -10.6441) ccw
  arc A252 (2.4185, -13.1054) -> (2.5302, -12.8128) centre (-2.4488, -11.0799) ccw
  arc A253 (2.5302, -12.8128) -> (2.9083, -12.8426) centre (4.2393, 6.4866) ccw
  arc A254 (2.9083, -12.8426) -> (2.9728, -13.149) centre (8.097, -11.9099) ccw
  arc A255 (2.9728, -13.149) -> (3.0771, -13.529) centre (9.2011, -11.6435) ccw
  arc A256 (3.0771, -13.529) -> (3.2349, -13.9888) centre (10.3287, -11.2968) ccw
  arc A257 (3.2349, -13.9888) -> (3.6341, -14.0044) centre (4.2393, 6.4866) ccw
  arc A258 (3.6341, -14.0044) -> (3.8275, -13.5585) centre (-3.2265, -10.7642) ccw
  arc A259 (3.8275, -13.5585) -> (3.9613, -13.1879) centre (-2.1297, -11.1983) ccw
  arc A260 (3.9613, -13.1879) -> (4.0497, -12.8874) centre (-1.0499, -11.5505) ccw
  arc A261 (4.0497, -12.8874) -> (4.4289, -12.8874) centre (4.2393, 6.4866) ccw
  arc A262 (4.4289, -12.8874) -> (4.5173, -13.1879) centre (9.5285, -11.5505) ccw
  arc A263 (4.5173, -13.1879) -> (4.6511, -13.5585) centre (10.6083, -11.1983) ccw
  arc A264 (4.6511, -13.5585) -> (4.8445, -14.0044) centre (11.7052, -10.7642) ccw
  arc A265 (4.8445, -14.0044) -> (5.2437, -13.9888) centre (4.2393, 6.4866) ccw
  arc A266 (5.2437, -13.9888) -> (5.4015, -13.529) centre (-1.85, -11.2968) ccw
  arc A267 (5.4015, -13.529) -> (5.5058, -13.149) centre (-0.7225, -11.6435) ccw
  arc A268 (5.5058, -13.149) -> (5.5703, -12.8426) centre (0.3816, -11.9099) ccw
  arc A269 (5.5703, -12.8426) -> (5.9484, -12.8128) centre (4.2393, 6.4866) ccw
  arc A270 (5.9484, -12.8128) -> (6.0601, -13.1054) centre (10.9274, -11.0799) ccw
  arc A271 (6.0601, -13.1054) -> (6.2226, -13.4644) centre (11.9762, -10.6441) ccw
  arc A272 (6.2226, -13.4644) -> (6.4504, -13.8938) centre (13.0356, -10.1253) ccw
  arc A273 (6.4504, -13.8938) -> (6.8471, -13.8468) centre (4.2393, 6.4866) ccw
  arc A274 (6.8471, -13.8468) -> (6.9683, -13.3761) centre (-0.436, -11.7197) ccw
  arc A275 (6.9683, -13.3761) -> (7.0425, -12.9891) centre (0.7152, -11.9769) ccw
  arc A276 (7.0425, -12.9891) -> (7.0828, -12.6786) centre (1.8368, -12.1558) ccw
  arc A277 (7.0828, -12.6786) -> (7.4574, -12.6193) centre (4.2393, 6.4866) ccw
  arc A278 (7.4574, -12.6193) -> (7.5917, -12.9022) centre (12.285, -10.501) ccw
  arc A279 (7.5917, -12.9022) -> (7.7818, -13.2473) centre (13.2964, -9.9842) ccw
  arc A280 (7.7818, -13.2473) -> (8.0426, -13.6575) centre (14.3119, -9.3839) ccw
  arc A281 (8.0426, -13.6575) -> (8.4344, -13.5796) centre (4.2393, 6.4866) ccw
  arc A282 (8.4344, -13.5796) -> (8.5183, -13.1007) centre (1.0069, -12.0304) ccw
  arc A283 (8.5183, -13.1007) -> (8.5619, -12.7092) centre (2.1747, -12.1965) ccw
  arc A284 (8.5619, -12.7092) -> (8.5777, -12.3964) centre (3.3069, -12.2869) ccw
  arc A285 (8.5777, -12.3964) -> (8.9465, -12.3079) centre (4.2393, 6.4866) ccw
  arc A286 (8.9465, -12.3079) -> (9.1026, -12.5794) centre (13.5931, -9.8174) ccw
  arc A287 (9.1026, -12.5794) -> (9.3192, -12.9085) centre (14.5608, -9.2228) ccw
  arc A288 (9.3192, -12.9085) -> (9.6113, -13.297) centre (15.526, -8.5447) ccw
  arc A289 (9.6113, -13.297) -> (9.9958, -13.1886) centre (4.2393, 6.4866) ccw
  arc A290 (9.9958, -13.1886) -> (10.0419, -12.7046) centre (2.4697, -12.227) ccw
  arc A291 (10.0419, -12.7046) -> (10.0547, -12.3109) centre (3.647, -12.3009) ccw
  arc A292 (10.0547, -12.3109) -> (10.0459, -11.9978) centre (4.7827, -12.3021) ccw
  arc A293 (10.0459, -11.9978) -> (10.4066, -11.8806) centre (4.2393, 6.4866) ccw
  arc A294 (10.4066, -11.8806) -> (10.5835, -12.139) centre (14.8434, -9.0332) ccw
  arc A295 (10.5835, -12.139) -> (10.8252, -12.4501) centre (15.7615, -8.3646) ccw
  arc A296 (10.8252, -12.4501) -> (11.147, -12.8145) centre (16.6706, -7.6128) ccw
  arc A297 (11.147, -12.8145) -> (11.5218, -12.6763) centre (4.2393, 6.4866) ccw
  arc A298 (11.5218, -12.6763) -> (11.5298, -12.1902) centre (3.9434, -12.3081) ccw
  arc A299 (11.5298, -12.1902) -> (11.5116, -11.7966) centre (5.1228, -12.2894) ccw
  arc A300 (11.5116, -11.7966) -> (11.4783, -11.4853) centre (6.2552, -12.2016) ccw
  arc A301 (11.4783, -11.4853) -> (11.8286, -11.3401) centre (4.2393, 6.4866) ccw
  arc A302 (11.8286, -11.3401) -> (12.0253, -11.5839) centre (16.0284, -8.1534) ccw
  arc A303 (12.0253, -11.5839) -> (12.2907, -11.875) centre (16.8912, -7.4148) ccw
  arc A304 (12.2907, -11.875) -> (12.64, -12.213) centre (17.7385, -6.594) ccw
  arc A305 (12.64, -12.213) -> (13.0028, -12.0458) centre (4.2393, 6.4866) ccw
  arc A306 (13.0028, -12.0458) -> (12.9727, -11.5606) centre (5.4189, -12.2734) ccw
  arc A307 (12.9727, -11.5606) -> (12.9236, -11.1697) centre (6.5933, -12.1622) ccw
  arc A308 (12.9236, -11.1697) -> (12.866, -10.8619) centre (7.7153, -11.9858) ccw
  arc A309 (12.866, -10.8619) -> (13.2039, -10.6897) centre (4.2393, 6.4866) ccw
  arc A310 (13.2039, -10.6897) -> (13.4191, -10.9173) centre (17.1407, -7.1833) ccw
  arc A311 (13.4191, -10.9173) -> (13.7065, -11.1867) centre (17.9429, -6.3793) ccw
  arc A312 (13.7065, -11.1867) -> (14.0813, -11.4963) centre (18.7231, -5.4945) ccw
  arc A313 (14.0813, -11.4963) -> (14.4298, -11.3011) centre (4.2393, 6.4866) ccw
  arc A314 (14.4298, -11.3011) -> (14.3617, -10.8198) centre (6.8872, -12.123) ccw
  arc A315 (14.3617, -10.8198) -> (14.2822, -10.4339) centre (8.0492, -11.92) ccw
  arc A316 (14.2822, -10.4339) -> (14.2006, -10.1316) centre (9.1539, -11.6561) ccw
  arc A317 (14.2006, -10.1316) -> (14.5239, -9.9334) centre (4.2393, 6.4866) ccw
  arc A318 (14.5239, -9.9334) -> (14.7563, -10.1434) centre (18.1735, -6.1289) ccw
  arc A319 (14.7563, -10.1434) -> (15.064, -10.3895) centre (18.9101, -5.2644) ccw
  arc A320 (15.064, -10.3895) -> (15.4619, -10.6687) centre (19.6185, -4.3212) ccw
  arc A321 (15.4619, -10.6687) -> (15.794, -10.4467) centre (4.2393, 6.4866) ccw
  arc A322 (15.794, -10.4467) -> (15.6884, -9.9722) centre (8.3391, -11.8579) ccw
  arc A323 (15.6884, -9.9722) -> (15.5788, -9.5938) centre (9.4816, -11.5644) ccw
  arc A324 (15.5788, -9.5938) -> (15.4737, -9.2988) centre (10.5622, -11.2146) ccw
  arc A325 (15.4737, -9.2988) -> (15.7805, -9.0759) centre (4.2393, 6.4866) ccw
  arc A326 (15.7805, -9.0759) -> (16.0286, -9.267) centre (19.1203, -4.9968) ccw
  arc A327 (16.0286, -9.267) -> (16.3547, -9.4881) centre (19.7869, -4.0772) ccw
  arc A328 (16.3547, -9.4881) -> (16.7733, -9.7353) centre (20.4191, -3.0813) ccw
  arc A329 (16.7733, -9.7353) -> (17.087, -9.488) centre (4.2393, 6.4866) ccw
  arc A330 (17.087, -9.488) -> (16.9444, -9.0232) centre (9.7657, -11.4797) ccw
  arc A331 (16.9444, -9.0232) -> (16.8055, -8.6545) centre (10.8817, -11.0974) ccw
  arc A332 (16.8055, -8.6545) -> (16.6776, -8.3687) centre (11.9315, -10.664) ccw
  arc A333 (16.6776, -8.3687) -> (16.966, -8.1224) centre (4.2393, 6.4866) ccw
  arc A334 (16.966, -8.1224) -> (17.2283, -8.2934) centre (19.9754, -3.7938) ccw
  arc A335 (17.2283, -8.2934) -> (17.5707, -8.4883) centre (20.5678, -2.8247) ccw
  arc A336 (17.5707, -8.4883) -> (18.0074, -8.7019) centre (21.1199, -1.7823) ccw
  arc A337 (18.0074, -8.7019) -> (18.3007, -8.4307) centre (4.2393, 6.4866) ccw
  arc A338 (18.3007, -8.4307) -> (18.1221, -7.9786) centre (11.1583, -10.9907) ccw
  arc A339 (18.1221, -7.9786) -> (17.9547, -7.6219) centre (12.2409, -10.5221) ccw
  arc A340 (17.9547, -7.6219) -> (17.8048, -7.347) centre (13.2534, -10.0076) ccw
  arc A341 (17.8048, -7.347) -> (18.0729, -7.0788) centre (4.2393, 6.4866) ccw
  arc A342 (18.0729, -7.0788) -> (18.3479, -7.2288) centre (20.7335, -2.5275) ccw
  arc A343 (18.3479, -7.2288) -> (18.7045, -7.3962) centre (21.248, -1.5149) ccw
  arc A344 (18.7045, -7.3962) -> (19.1566, -7.5748) centre (21.7166, -0.4324) ccw
  arc A345 (19.1566, -7.5748) -> (19.4278, -7.2815) centre (4.2393, 6.4866) ccw
  arc A346 (19.4278, -7.2815) -> (19.2143, -6.8447) centre (12.5083, -10.394) ccw
  arc A347 (19.2143, -6.8447) -> (19.0194, -6.5023) centre (13.5507, -9.8418) ccw
  arc A348 (19.0194, -6.5023) -> (18.8483, -6.24) centre (14.5198, -9.2495) ccw
  arc A349 (18.8483, -6.24) -> (19.0946, -5.9516) centre (4.2393, 6.4866) ccw
  arc A350 (19.0946, -5.9516) -> (19.3805, -6.0795) centre (21.3899, -1.2056) ccw
  arc A351 (19.3805, -6.0795) -> (19.7492, -6.2185) centre (21.8234, -0.1558) ccw
  arc A352 (19.7492, -6.2185) -> (20.2139, -6.3611) centre (22.2056, 0.9602) ccw
  arc A353 (20.2139, -6.3611) -> (20.4612, -6.0473) centre (4.2393, 6.4866) ccw
  arc A354 (20.4612, -6.0473) -> (20.2141, -5.6287) centre (13.8072, -9.6932) ccw
  arc A355 (20.2141, -5.6287) -> (19.9929, -5.3027) centre (14.8031, -9.0609) ccw
  arc A356 (19.9929, -5.3027) -> (19.8018, -5.0546) centre (15.7227, -8.3944) ccw
  arc A357 (19.8018, -5.0546) -> (20.0247, -4.7478) centre (4.2393, 6.4866) ccw
  arc A358 (20.0247, -4.7478) -> (20.3197, -4.8528) centre (21.9406, 0.1637) ccw
  arc A359 (20.3197, -4.8528) -> (20.6982, -4.9624) centre (22.2903, 1.2443) ccw
  arc A360 (20.6982, -4.9624) -> (21.1727, -5.0681) centre (22.5838, 2.3868) ccw
  arc A361 (21.1727, -5.0681) -> (21.3946, -4.736) centre (4.2393, 6.4866) ccw
  arc A362 (21.3946, -4.736) -> (21.1154, -4.338) centre (15.0472, -8.8926) ccw
  arc A363 (21.1154, -4.338) -> (20.8693, -4.0303) centre (15.9904, -8.1842) ccw
  arc A364 (20.8693, -4.0303) -> (20.6593, -3.798) centre (16.8549, -7.4475) ccw
  arc A365 (20.6593, -3.798) -> (20.8575, -3.4746) centre (4.2393, 6.4866) ccw
  arc A366 (20.8575, -3.4746) -> (21.1598, -3.5562) centre (22.3821, 1.5721) ccw
  arc A367 (21.1598, -3.5562) -> (21.5457, -3.6358) centre (22.646, 2.6768) ccw
  arc A368 (21.5457, -3.6358) -> (22.027, -3.7039) centre (22.8489, 3.8388) ccw
  arc A369 (22.027, -3.7039) -> (22.2222, -3.3554) centre (4.2393, 6.4866) ccw
  arc A370 (22.2222, -3.3554) -> (21.9127, -2.9806) centre (16.2205, -7.9972) ccw
  arc A371 (21.9127, -2.9806) -> (21.6432, -2.6931) centre (17.1052, -7.217) ccw
  arc A372 (21.6432, -2.6931) -> (21.4156, -2.478) centre (17.9092, -6.4148) ccw
  arc A373 (21.4156, -2.478) -> (21.5878, -2.1401) centre (4.2393, 6.4866) ccw
  arc A374 (21.5878, -2.1401) -> (21.8956, -2.1977) centre (22.7117, 3.0107) ccw
  arc A375 (21.8956, -2.1977) -> (22.2866, -2.2467) centre (22.8881, 4.1327) ccw
  arc A376 (22.2866, -2.2467) -> (22.7717, -2.2769) centre (22.9993, 5.307) ccw
  arc A377 (22.7717, -2.2769) -> (22.939, -1.9141) centre (4.2393, 6.4866) ccw
  arc A378 (22.939, -1.9141) -> (22.601, -1.5647) centre (17.3199, -7.0125) ccw
  arc A379 (22.601, -1.5647) -> (22.3098, -1.2993) centre (18.1407, -6.1653) ccw
  arc A380 (22.3098, -1.2993) -> (22.0661, -1.1027) centre (18.8793, -5.3025) ccw
  arc A381 (22.0661, -1.1027) -> (22.2112, -0.7523) centre (4.2393, 6.4866) ccw
  arc A382 (22.2112, -0.7523) -> (22.5226, -0.7856) centre (22.9275, 4.4707) ccw
  arc A383 (22.5226, -0.7856) -> (22.9161, -0.8038) centre (23.0153, 5.6031) ccw
  arc A384 (22.9161, -0.8038) -> (23.4022, -0.7958) centre (23.034, 6.7826) ccw
  arc A385 (23.4022, -0.7958) -> (23.5404, -0.4211) centre (4.2393, 6.4866) ccw
  arc A386 (23.5404, -0.4211) -> (23.1761, -0.0993) centre (18.3387, -5.9446) ccw
  arc A387 (23.1761, -0.0993) -> (22.865, 0.1425) centre (19.0905, -5.0356) ccw
  arc A388 (22.865, 0.1425) -> (22.6065, 0.3194) centre (19.7592, -4.1175) ccw
  arc A389 (22.6065, 0.3194) -> (22.7237, 0.6801) centre (4.2393, 6.4866) ccw
  arc A390 (22.7237, 0.6801) -> (23.0368, 0.6713) centre (23.0281, 5.9432) ccw
  arc A391 (23.0368, 0.6713) -> (23.4306, 0.684) centre (23.0268, 7.079) ccw
  arc A392 (23.4306, 0.684) -> (23.9145, 0.7301) centre (22.9529, 8.2563) ccw
  arc A393 (23.9145, 0.7301) -> (24.0229, 1.1146) centre (4.2393, 6.4866) ccw
  arc A394 (24.0229, 1.1146) -> (23.6344, 1.4068) centre (19.2706, -4.8001) ccw
  arc A395 (23.6344, 1.4068) -> (23.3053, 1.6234) centre (19.9488, -3.8349) ccw
  arc A396 (23.3053, 1.6234) -> (23.0338, 1.7794) centre (20.5433, -2.8671) ccw
  arc A397 (23.0338, 1.7794) -> (23.1223, 2.1482) centre (4.2393, 6.4866) ccw
  arc A398 (23.1223, 2.1482) -> (23.4351, 2.164) centre (23.0128, 7.419) ccw
  arc A399 (23.4351, 2.164) -> (23.8267, 2.2076) centre (22.9224, 8.5512) ccw
  arc A400 (23.8267, 2.2076) -> (24.3055, 2.2916) centre (22.7564, 9.7191) ccw
  arc A401 (24.3055, 2.2916) -> (24.3834, 2.6834) centre (4.2393, 6.4866) ccw
  arc A402 (24.3834, 2.6834) -> (23.9732, 2.9442) centre (20.1098, -3.5859) ccw
  arc A403 (23.9732, 2.9442) -> (23.6281, 3.1343) centre (20.7102, -2.5705) ccw
  arc A404 (23.6281, 3.1343) -> (23.3452, 3.2686) centre (21.2269, -1.5591) ccw
  arc A405 (23.3452, 3.2686) -> (23.4045, 3.6431) centre (4.2393, 6.4866) ccw
  arc A406 (23.4045, 3.6431) -> (23.7151, 3.6834) centre (22.8818, 8.8891) ccw
  arc A407 (23.7151, 3.6834) -> (24.102, 3.7576) centre (22.7028, 10.0107) ccw
  arc A408 (24.102, 3.7576) -> (24.5728, 3.8789) centre (22.4457, 11.1619) ccw
  arc A409 (24.5728, 3.8789) -> (24.6197, 4.2756) centre (4.2393, 6.4866) ccw
  arc A410 (24.6197, 4.2756) -> (24.1903, 4.5034) centre (20.8512, -2.3097) ccw
  arc A411 (24.1903, 4.5034) -> (23.8314, 4.6658) centre (21.37, -1.2503) ccw
  arc A412 (23.8314, 4.6658) -> (23.5388, 4.7775) centre (21.8058, -0.2015) ccw
  arc A413 (23.5388, 4.7775) -> (23.5685, 5.1556) centre (4.2393, 6.4866) ccw
  arc A414 (23.5685, 5.1556) -> (23.875, 5.2201) centre (22.6358, 10.3443) ccw
  arc A415 (23.875, 5.2201) -> (24.2549, 5.3244) centre (22.3694, 11.4485) ccw
  arc A416 (24.2549, 5.3244) -> (24.7147, 5.4823) centre (22.0227, 12.576) ccw
  arc A417 (24.7147, 5.4823) -> (24.7304, 5.8814) centre (4.2393, 6.4866) ccw
  arc A418 (24.7304, 5.8814) -> (24.2844, 6.0748) centre (21.4901, -0.9792) ccw
  arc A419 (24.2844, 6.0748) -> (23.9138, 6.2086) centre (21.9242, 0.1176) ccw
  arc A420 (23.9138, 6.2086) -> (23.6134, 6.297) centre (22.2764, 1.1974) ccw
  arc A421 (23.6134, 6.297) -> (23.6134, 6.6762) centre (4.2393, 6.4866) ccw
  arc A422 (23.6134, 6.6762) -> (23.9138, 6.7646) centre (22.2764, 11.7758) ccw
  arc A423 (23.9138, 6.7646) -> (24.2844, 6.8984) centre (21.9242, 12.8556) ccw
  arc A424 (24.2844, 6.8984) -> (24.7304, 7.0918) centre (21.4901, 13.9525) ccw
  arc A425 (24.7304, 7.0918) -> (24.7147, 7.491) centre (4.2393, 6.4866) ccw
  arc A426 (24.7147, 7.491) -> (24.2549, 7.6488) centre (22.0227, 0.3973) ccw
  arc A427 (24.2549, 7.6488) -> (23.875, 7.7531) centre (22.3694, 1.5248) ccw
  arc A428 (23.875, 7.7531) -> (23.5685, 7.8177) centre (22.6358, 2.6289) ccw
  arc A429 (23.5685, 7.8177) -> (23.5388, 8.1957) centre (4.2393, 6.4866) ccw
  arc A430 (23.5388, 8.1957) -> (23.8314, 8.3074) centre (21.8058, 13.1747) ccw
  arc A431 (23.8314, 8.3074) -> (24.1903, 8.4699) centre (21.37, 14.2235) ccw
  arc A432 (24.1903, 8.4699) -> (24.6197, 8.6977) centre (20.8512, 15.2829) ccw
  arc A433 (24.6197, 8.6977) -> (24.5728, 9.0944) centre (4.2393, 6.4866) ccw
  arc A434 (24.5728, 9.0944) -> (24.102, 9.2156) centre (22.4457, 1.8113) ccw
  arc A435 (24.102, 9.2156) -> (23.7151, 9.2898) centre (22.7028, 2.9626) ccw
  arc A436 (23.7151, 9.2898) -> (23.4045, 9.3301) centre (22.8818, 4.0842) ccw
  arc A437 (23.4045, 9.3301) -> (23.3452, 9.7047) centre (4.2393, 6.4866) ccw
  arc A438 (23.3452, 9.7047) -> (23.6281, 9.839) centre (21.2269, 14.5323) ccw
  arc A439 (23.6281, 9.839) -> (23.9732, 10.0291) centre (20.7102, 15.5438) ccw
  arc A440 (23.9732, 10.0291) -> (24.3834, 10.2899) centre (20.1098, 16.5592) ccw
  arc A441 (24.3834, 10.2899) -> (24.3055, 10.6817) centre (4.2393, 6.4866) ccw
  arc A442 (24.3055, 10.6817) -> (23.8267, 10.7656) centre (22.7564, 3.2542) ccw
  arc A443 (23.8267, 10.7656) -> (23.4351, 10.8092) centre (22.9224, 4.422) ccw
  arc A444 (23.4351, 10.8092) -> (23.1223, 10.825) centre (23.0128, 5.5542) ccw
  arc A445 (23.1223, 10.825) -> (23.0338, 11.1938) centre (4.2393, 6.4866) ccw
  arc A446 (23.0338, 11.1938) -> (23.3053, 11.3499) centre (20.5433, 15.8404) ccw
  arc A447 (23.3053, 11.3499) -> (23.6344, 11.5665) centre (19.9488, 16.8081) ccw
  arc A448 (23.6344, 11.5665) -> (24.0229, 11.8587) centre (19.2706, 17.7733) ccw
  arc A449 (24.0229, 11.8587) -> (23.9145, 12.2431) centre (4.2393, 6.4866) ccw
  arc A450 (23.9145, 12.2431) -> (23.4306, 12.2893) centre (22.9529, 4.717) ccw
  arc A451 (23.4306, 12.2893) -> (23.0368, 12.302) centre (23.0268, 5.8943) ccw
  arc A452 (23.0368, 12.302) -> (22.7237, 12.2932) centre (23.0281, 7.0301) ccw
  arc A453 (22.7237, 12.2932) -> (22.6065, 12.6539) centre (4.2393, 6.4866) ccw
  arc A454 (22.6065, 12.6539) -> (22.865, 12.8308) centre (19.7592, 17.0907) ccw
  arc A455 (22.865, 12.8308) -> (23.1761, 13.0725) centre (19.0905, 18.0089) ccw
  arc A456 (23.1761, 13.0725) -> (23.5404, 13.3943) centre (18.3387, 18.9179) ccw
  arc A457 (23.5404, 13.3943) -> (23.4022, 13.7691) centre (4.2393, 6.4866) ccw
  arc A458 (23.4022, 13.7691) -> (22.9161, 13.7771) centre (23.034, 6.1907) ccw
  arc A459 (22.9161, 13.7771) -> (22.5226, 13.7589) centre (23.0153, 7.3701) ccw
  arc A460 (22.5226, 13.7589) -> (22.2112, 13.7256) centre (22.9275, 8.5025) ccw